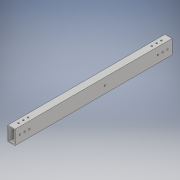
# Autodesk Inventor part: nhk17
Saved by Autodesk Inventor 2019 (Build 230136000, 136)
## iProperties
Created: 2022-02-15
Part Number: nhk17
Material: 一般
Document SubType Name: Sheet Metal
Designer: yuta
Density: 1 g/cm^3
Sheet Metal Rule: Default_mm
Appearance: 既定
Author: yuta
Autodesk Inventor part; units mm, degrees
ref_plane "YZ Plane" through (0, 0, 0) normal (1, 0, 0) x (0, 1, 0)
ref_plane "XZ Plane" through (0, 0, 0) normal (0, 1, 0) x (-1, 0, 0)
ref_plane "XY Plane" through (0, 0, 0) normal (0, 0, 1) x (1, 0, 0)
sketch "スケッチ1" plane through (0, 0, 0) normal (0, 0, 1) x (1, 0, 0)
  line L0 (-11.3154, 7.0975) -> (3.6846, 7.0975)
  line L1 (3.6846, 7.0975) -> (3.6846, -22.9025)
  line L2 (3.6846, -22.9025) -> (-11.3154, -22.9025)
  line L3 (-11.3154, -22.9025) -> (-11.3154, 7.0975)
  point P0 (0, 0)
  dimension "d0" = 15
  dimension "d1" = 30
  constraints: 8 end point, 2 parallel, 1 horizontal, 1 perpendicular
  measures "d0" distance of L1.end L2.end
  measures "d1" distance of L0.end L1.end
extrude "押し出し1" add sketch "スケッチ1" along normal blind 330
sketch "スケッチ2" plane through (3.6846, -22.9025, 0) normal (1, 0, 0) x (0, 0, -1)
  circle A0 centre (-320, 15) radius 1.5
  line L0 (0, 30) -> (-330, 30) projected
  line L1 (-330, 0) -> (-330, 30) projected
  circle A1 centre (-310, 15) radius 1.5
  circle A2 centre (-300, 15) radius 1.5
  circle A3 centre (-30, 15) radius 1.5
  circle A4 centre (-20, 15) radius 1.5
  circle A5 centre (-10, 15) radius 1.5
  line L2 (0, 30) -> (0, 0) projected
  point P0 (0, 22.9025)
  dimension "d4" = 3
  dimension "d5" = 15
  dimension "d6" = 10
  dimension "d7" = 3
  dimension "d8" = 3
  dimension "d9" = 3
  dimension "d10" = 3
  dimension "d11" = 3
  dimension "d12" = 10
  dimension "d13" = 10
  dimension "d14" = 10
  dimension "d15" = 10
  dimension "d16" = 10
  constraints: 6 centre point
  measures "d4" diameter of A0
  measures "d5" distance from line of L0 A0.centre
  measures "d6" distance from line of L1 A0.centre
  measures "d7" diameter of A1
  measures "d8" diameter of A2
  measures "d9" diameter of A3
  measures "d10" diameter of A4
  measures "d11" diameter of A5
  measures "d12" distance of A1.centre A0.centre
  measures "d13" distance of A2.centre A1.centre
  measures "d14" distance from line of A5.centre L2
  measures "d15" distance of A5.centre A4.centre
  measures "d16" distance of A4.centre A3.centre
hole "穴1" at (3.6846, -7.9025, 320) at (3.6846, -7.9025, 310) at (3.6846, -7.9025, 300) at (3.6846, -7.9025, 10) at (3.6846, -7.9025, 20) at (3.6846, -7.9025, 30) direction (-1, 0, 0) diameter 3 depth 15
sketch "スケッチ3" plane through (-11.3154, 7.0975, 0) normal (0, 1, 0) x (1, 0, 0)
  circle A0 centre (7.5, -15) radius 1.5
  line L0 (0, 0) -> (15, 0) projected
  circle A1 centre (7.5, -25) radius 1.5
  circle A2 centre (7.5, -35) radius 1.5
  circle A3 centre (7.5, -315) radius 1.5
  line L1 (15, -330) -> (0, -330) projected
  circle A4 centre (7.5, -305) radius 1.5
  circle A5 centre (7.5, -295) radius 1.5
  point P0 (11.3154, 0)
  dimension "d24" = 3
  dimension "d25" = 15
  dimension "d26" = 3
  dimension "d27" = 3
  dimension "d28" = 3
  dimension "d29" = 15
  dimension "d30" = 3
  dimension "d31" = 3
  dimension "d32" = 10
  dimension "d33" = 10
  dimension "d34" = 10
  dimension "d35" = 10
  constraints: 6 centre point
  measures "d24" diameter of A0
  measures "d25" distance from line of A0.centre L0
  measures "d26" diameter of A1
  measures "d27" diameter of A2
  measures "d28" diameter of A3
  measures "d29" distance from line of A3.centre L1
  measures "d30" diameter of A4
  measures "d31" diameter of A5
  measures "d32" distance of A1.centre A0.centre
  measures "d33" distance of A2.centre A1.centre
  measures "d34" distance of A4.centre A3.centre
  measures "d35" distance of A5.centre A4.centre
hole "穴2" at (-3.8154, 7.0975, 295) at (-3.8154, 7.0975, 305) at (-3.8154, 7.0975, 315) at (-3.8154, 7.0975, 15) at (-3.8154, 7.0975, 25) at (-3.8154, 7.0975, 35) direction (0, -1, 0) diameter 3 depth 30
sketch "スケッチ4" plane through (0, 0, 330) normal (0, 0, 1) x (1, 0, 0)
  line L0 (-9.8154, 5.5975) -> (2.1846, 5.5975)
  line L1 (2.1846, 5.5975) -> (2.1846, -21.4025)
  line L2 (2.1846, -21.4025) -> (-9.8154, -21.4025)
  line L3 (-9.8154, -21.4025) -> (-9.8154, 5.5975)
  line L4 (3.6846, 7.0975) -> (-11.3154, 7.0975) projected
  line L5 (-11.3154, 7.0975) -> (-11.3154, -22.9025) projected
  point P0 (0, 0)
  dimension "d43" = 12
  dimension "d44" = 27
  dimension "d45" = 1.5
  dimension "d46" = 1.5
  constraints: 8 end point, 2 parallel, 1 horizontal, 1 perpendicular
  measures "d43" distance of L1.end L2.end
  measures "d44" distance of L0.end L1.end
  measures "d45" distance between parallel lines of L0 L4
  measures "d46" distance between parallel lines of L3 L5
extrude "押し出し2" cut sketch "スケッチ4" against normal blind 330
sketch "スケッチ5" plane through (3.6846, -22.9025, 0) normal (1, 0, 0) x (0, 0, -1)
  circle A0 centre (-141, 15) radius 1.5
  line L0 (0, 30) -> (-330, 30) projected
  line L1 (0, 30) -> (0, 0) projected
  point P0 (0, 22.9025)
  dimension "d49" = 3
  dimension "d50" = 15
  dimension "d51" = 141
  constraints: 1 centre point
  measures "d49" diameter of A0
  measures "d50" distance from line of L0 A0.centre
  measures "d51" distance from line of L1 A0.centre
hole "穴3" at (3.6846, -7.9025, 141) direction (-1, 0, 0) diameter 3 depth 15
equation "\"BendRadius\" = Thickness"
equation "\"BendReliefWidth\" = Thickness"
equation "\"BendReliefDepth\" = 0.5 * Thickness"
equation "\"CornerReliefSize\" = 4 * Thickness"
equation "\"MinimumRemnant\" = 2 * Thickness"
equation "\"TransitionRadius\" = BendRadius"
equation "\"JacobiRadiusSize\" = BendRadius"
equation "\"GapSize\" = Thickness"
equation "\"Thickness\" = 0.5"
